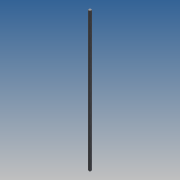
# Autodesk Inventor part: Gewindestange_M8x420mm
Saved by Autodesk Inventor 2015 SP1 (Build 190203100, 203)
## iProperties
Created: 2015-03-05
Part Number: Gewindestange_M8x420mm
Material: Generisch
Document SubType Name: Modeling
Designer: Marc
Density: 1 g/cm^3
Appearance: Vorgabe
Author: Marc
Autodesk Inventor part; units mm, degrees
ref_plane "YZ Plane" through (0, 0, 0) normal (1, 0, 0) x (0, 1, 0)
ref_plane "XZ Plane" through (0, 0, 0) normal (0, 1, 0) x (-1, 0, 0)
ref_plane "XY Plane" through (0, 0, 0) normal (0, 0, 1) x (1, 0, 0)
sketch "Skizze1" plane through (0, 0, 0) normal (0, 0, 1) x (1, 0, 0)
  line L0 (-5.6, 0) -> (5.6, 0) projected
  line L1 (0, -5.6) -> (0, 5.6) projected
  circle A0 centre (0, 0) radius 4
  dimension "d0" = 8
  constraints: 1 centre point, 1 coincident
  measures "d0" diameter of A0
extrude "Extrusion1" add sketch "Skizze1" along normal blind 420
thread "Gewinde1" size "M8x1.25" class "6g" standard "ANSI Metric M Profile" full length
chamfer "Fase1" distance 0.5 angle 45 1 edges at (-4, 0, 420)
chamfer "Fase2" distance 0.5 angle 45 1 edges at (-4, 0, 0)
